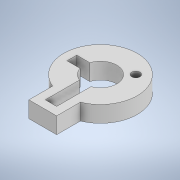
# Autodesk Inventor part: Pièce_maintient_pièce
Saved by Autodesk Inventor 2020.1 (Build 241239000, 239)
## iProperties
Created: 2019-08-23
Part Number: Pièce_maintient_pièce
Material: Générique
Document SubType Name: Modeling
Designer: marlo
Density: 1 g/cm^3
Appearance: Par défaut
Author: marlo
Autodesk Inventor part; units mm, degrees
ref_plane "YZ Plane" through (0, 0, 0) normal (1, 0, 0) x (0, 1, 0)
ref_plane "XZ Plane" through (0, 0, 0) normal (0, 1, 0) x (-1, 0, 0)
ref_plane "XY Plane" through (0, 0, 0) normal (0, 0, 1) x (1, 0, 0)
sketch "Esquisse1" plane through (0, 0, 0) normal (0, 1, 0) x (-1, 0, 0)
  circle A0 centre (-0.3398, 0) radius 22.5
  circle A1 centre (-0.3398, 0) radius 10
  line L0 (3.1602, 9.3675) -> (-3.8398, 9.3675)
  line L1 (-3.8398, 9.3675) -> (-3.8398, 30.3675)
  line L2 (-3.8398, 30.3675) -> (3.1602, 30.3675)
  line L3 (3.1602, 30.3675) -> (3.1602, 9.3675)
  line L4 (-8.8398, 35.3675) -> (-8.8398, 4.3675)
  line L5 (-8.8398, 4.3675) -> (8.1602, 4.3675)
  line L6 (8.1602, 4.3675) -> (8.1602, 35.3675)
  line L7 (8.1602, 35.3675) -> (-8.8398, 35.3675)
  line L8 (17.1996, -3) -> (9.1996, -3)
  line L9 (9.1996, -3) -> (9.1996, 3)
  line L10 (9.1996, 3) -> (17.1996, 3)
  line L11 (17.1996, 3) -> (17.1996, -3)
  line L12 (15.5701, 15.9099) -> (-16.2497, -15.9099) construction
  line L13 (-0.3398, -15.9099) -> (-16.2497, -15.9099) construction
  line L14 (-16.2497, -15.9099) -> (-16.2497, 0) construction
  line L15 (-0.3398, -15.9099) -> (-0.3398, 0) construction
  line L16 (-0.3398, 0) -> (-16.2497, 0) construction
  circle A2 centre (-11.1699, -10.8301) radius 2.5
  line L17 (-11.1699, -10.8301) -> (-16.2497, -15.9099) construction
  line L18 (-7.4109, -7.0711) -> (-11.1699, -10.8301) construction
  point P0 (-8.8398, 20.8327)
  point P1 (8.1602, 20.8327)
  dimension "d2" = 45
  dimension "d3" = 20
  dimension "d4" = 7
  dimension "d5" = 21
  dimension "d6" = 5
  dimension "d7" = 6
  dimension "d8" = 8
  dimension "d9" = 5
  constraints: 38 end point, 7 point on circle, 6 parallel, 4 horizontal, 4 perpendicular, 3 centre point, 2 midpoint, 2 point on line, 2 vertical, 1 coincident, 3 other
  measures "d2" diameter of A0
  measures "d3" diameter of A1
  measures "d4" distance of L1.end L3.start
  measures "d5" distance of L3.start L0.start
  measures "d6" distance between parallel lines of L1 L4
  measures "d7" distance of L11.start L8.start
  measures "d8" distance of L8.start L9.start
  measures "d9" diameter of A2
extrude "Extrusion1" add sketch "Esquisse1" along normal blind 10 contours A0 L4 A1 L8 L11 L10 L6 | L6 A1 L3 A0 | A0 L3 L2 L1 L4 L7 L6 | A0 L1 A1 L4
chamfer "Chanfrein1" distance 2 distance2 1 1 edges at (13.6699, 0, -10.8301) measured on face at (8.7023, 6.6667, -11.2311)
